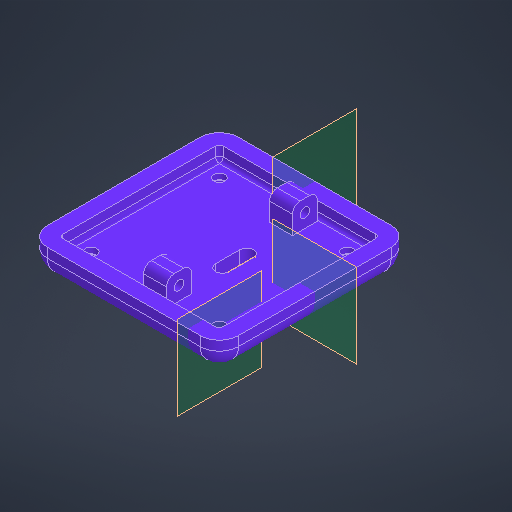
# Autodesk Inventor part: case2
Saved by Autodesk Inventor 2026.2 (Build 302298000, 298)
## iProperties
Created: 2025-11-11
Part Number: case2
Material: Generic
Document SubType Name: Modeling
Designer: micyg
Density: 1 g/cm^3
Appearance: Default
Author: micyg
Autodesk Inventor part; units mm, degrees
note: some values were not read from the file. Left out: dimensions or parameters whose unit could not be read.
ref_plane "YZ Plane" through (0, 0, 0) normal (1, 0, 0) x (0, 1, 0)
ref_plane "XZ Plane" through (0, 0, 0) normal (0, 1, 0) x (-1, 0, 0)
ref_plane "XY Plane" through (0, 0, 0) normal (0, 0, 1) x (1, 0, 0)
sketch "Sketch1" plane through (0, 0, 0) normal (0, 1, 0) x (-1, 0, 0)
  line L0 (0, 0) -> (50, 0)
  line L1 (50, 0) -> (50, -50)
  line L2 (50, -50) -> (0, -50)
  line L3 (0, -50) -> (0, 0)
  dimension "d0" = 50
  dimension "d1" = 50
  constraints: 8 end point, 2 parallel, 1 horizontal, 1 perpendicular
  measures "d0" distance of L1.end L2.end
  measures "d1" distance of L0.end L1.end
extrude "Extrusion1" add sketch "Sketch1" along normal blind 7.5
fillet "Fillet1" radius 5 4 edges at (-50, 3.75, 0) (-50, 3.75, -50) (0, 3.75, -50) (0, 3.75, 0)
ref_plane "Work Plane2" through (-25, 7.5, -50) normal (-1, 0, 0) x (0, -1, 0)
ref_plane "Work Plane1" through (0, 7.5, -25) normal (0, 0, -1) x (-1, 0, 0)
fillet "Fillet2" radius 5 8 edges at (-1.4645, 0, -48.5355) (-25, 0, -50) (-48.5355, 0, -48.5355) (-50, 0, -25) (-48.5355, 0, -1.4645) (-25, 0, 0) (-1.4645, 0, -1.4645) (0, 0, -25)
shell "Shell1" thickness 4 removed faces 1 at (-16.6667, 7.5, -18.3333)
sketch "Sketch2" plane through (0, 0, 0) normal (0, -1, 0) x (1, 0, 0)
  line L0 (-25, -60) -> (-25, 10) projected
  line L1 (10, -25) -> (-60, -25) projected
  line L2 (-8.2, -8.2) -> (-41.8, -8.2) construction
  line L3 (-41.8, -8.2) -> (-41.8, -41.8) construction
  line L4 (-41.8, -41.8) -> (-8.2, -41.8) construction
  line L5 (-8.2, -41.8) -> (-8.2, -8.2) construction
  circle A0 centre (-8.2, -8.2) radius 1.5
  point P0 (0, 0)
  point P1 (-5, -45)
  point P2 (-45, -45)
  point P3 (-25, -41.8)
  point P4 (-8.2, -25)
  point P5 (-8.2, -25)
  point P6 (-25, -41.8)
  dimension "d8" = 33.6
  dimension "d9" = 33.6
  dimension "d10" = 3
  constraints: 8 end point, 4 point on line, 2 midpoint, 2 parallel, 1 centre point, 1 coincident, 1 horizontal, 1 perpendicular
  measures "d8" distance of L4.end L2.start
  measures "d9" distance of L3.end L4.end
  measures "d10" diameter of A0
extrude "Extrusion2" cut sketch "Sketch2" against normal up to surface (4 mm away)
ref_plane "Work Plane3" through (-8.2, 0, -8.2) normal (-1, 0, 0) x (0, -1, 0)
sketch "Sketch3" plane through (-8.2, 0, -8.2) normal (-1, 0, 0) x (0, -1, 0)
  line L0 (-4, -1.5) -> (-4, 1.5) projected
  line L1 (0, 1.5) -> (0, -1.5) projected
  line L2 (0, -36.8) -> (0, 3.2) projected
  line L3 (0, 2.75) -> (-1.5, 2.75)
  line L4 (-1.5, 2.75) -> (-1.5, -2.75)
  line L5 (-1.5, -2.75) -> (0, -2.75)
  line L6 (0, -2.75) -> (0, 2.75)
  line L7 (-1.5, -2.75) -> (-2.5, -1.5)
  line L8 (0, -1.5) -> (-4, -1.5) projected
  line L9 (0, 0) -> (-4, 0)
  point P0 (0, 8.2)
  point P1 (0, -2.75)
  dimension "d13" = 5.5
  dimension "d14" = 1.5
  dimension "d15" = 1
  constraints: 12 end point, 3 midpoint, 2 parallel, 2 point on line, 1 horizontal, 1 perpendicular
  measures "d13" distance of L3.end L4.end
  measures "d14" distance of L4.end L5.end
  measures "d15" distance from line of L4 L7.end
revolve "Revolution1" cut sketch "Sketch3" angle 360 about axis through (-8.2, 0, -8.2) along (0, 1, 0) contours L8 L4 L7 | L4 L8 L2 L5
mirror "Mirror1" about plane through (0, 7.5, -25) normal (0, 0, -1) of "Extrusion2", "Revolution1"
mirror "Mirror2" about plane through (-25, 7.5, -50) normal (-1, 0, 0) of "Extrusion2", "Mirror1", "Revolution1"
sketch "Sketch4" plane through (-45, 4, -45) normal (0, 1, 0) x (1, 0, 0)
  line L0 (20, -55) -> (20, 15) construction
  line L1 (-15, -20) -> (55, -20) construction
  line L2 (24, -23.2) -> (24, -16.8) construction
  line L3 (25.8, -23.2) -> (25.8, -16.8)
  line L4 (22.2, -16.8) -> (22.2, -23.2)
  arc A0 (22.2, -23.2) -> (25.8, -23.2) centre (24, -23.2) ccw
  arc A1 (25.8, -16.8) -> (22.2, -16.8) centre (24, -16.8) ccw
  point P0 (45, -45)
  point P1 (24, -20)
  point P2 (24, -15)
  point P3 (24, -25)
  dimension "d17" = 3.6
  dimension "d38" = 6.4
  dimension "d39" = 4
  constraints: 8 end point, 6 point on circle, 4 tangent, 2 centre point, 2 parallel, 1 midpoint, 1 point on line
  measures "d17" distance between parallel lines of L3 L4
  measures "d38" distance of L2.start L2.end
  measures "d39" distance between parallel lines of L2 L0
extrude "Extrusion3" cut sketch "Sketch4" against normal up to surface (4 mm away)
ref_plane "Płaszczyzna konstrukcyjna9" through (-19.09, 4, -28.2) normal (-1, 0, 0) x (0, 0, 1)
sketch "Szkic6" plane through (-19.09, 4, -28.2) normal (-1, 0, 0) x (0, 0, 1)
  line L0 (0, 0) -> (0, 0) projected
  line L1 (0, 0) -> (6.4, 0) projected
  line L2 (6.4, 0) -> (6.4, 0) projected
  line L3 (6.4, 0) -> (0, 0) projected
  line L4 (-15.1, 0) -> (-12.1, 0) projected
  line L5 (18.5, 0) -> (21.5, 0) projected
  line L6 (-15.1, 0) -> (-12.1, 0) projected
  line L7 (18.5, 0) -> (21.5, 0) projected
  line L8 (23.2, 0) -> (-16.8, 0) projected
  line L9 (-16.8, 0) -> (23.2, 0) projected
  line L10 (6.4, -4) -> (6.4, -4) projected
  line L11 (6.4, 0) -> (6.4, -4) projected
  line L12 (6.4, 0) -> (6.4, 0) projected
  line L13 (6.4, 0) -> (6.4, -4) projected
  line L14 (0, -4) -> (0, -4) projected
  line L15 (0, 0) -> (0, -4) projected
  line L16 (0, 0) -> (0, 0) projected
  line L17 (0, 0) -> (0, -4) projected
  line L18 (-16.55, 0) -> (-10.05, 0)
  line L19 (-10.05, 0) -> (-10.05, 6.85)
  line L20 (-10.05, 6.85) -> (-16.55, 6.85)
  line L21 (-16.55, 6.85) -> (-16.55, 0)
  circle A0 centre (-13.3, 3.6) radius 1.25
  line L22 (-13.3, 0) -> (-13.3, 6.85) construction
  line L23 (3.2, -6.17) -> (3.2, 9.02) construction
  line L24 (22.95, 0) -> (16.45, 0)
  line L25 (16.45, 0) -> (16.45, 6.85)
  line L26 (16.45, 6.85) -> (22.95, 6.85)
  line L27 (22.95, 6.85) -> (22.95, 0)
  circle A1 centre (19.7, 3.6) radius 1.25
  line L28 (19.7, 0) -> (19.7, 6.85) construction
  point P0 (28.2, -4)
  point P1 (16.45, 0)
  point P2 (18.5, 0)
  point P3 (21.5, 0)
  point P4 (-16.55, 0)
  point P5 (-15.1, 0)
  point P6 (-12.1, 0)
  point P7 (-10.05, 0)
  dimension "d30" = 2
  dimension "d31" = 2
  dimension "d33" = 3.6
  dimension "d34" = 2.5
  dimension "d35" = 33
  constraints: 20 end point, 7 symmetric about line, 3 point on line, 2 centre point, 2 midpoint, 2 parallel, 1 horizontal, 1 perpendicular, 1 other
  measures "d30" distance edge to line of A0 L19
  measures "d31" distance edge to line of A0 L20
  measures "d33" distance from line of L8 A0.centre
  measures "d34" diameter of A0
  measures "d35" distance between parallel lines of L28 L22
extrude "Wyciągnięcie proste5" add sketch "Szkic6" along normal blind 6
fillet "Zaokrąglenie3" radius 2 4 edges at (-22.09, 10.85, -38.25) (-22.09, 10.85, -44.75) (-22.09, 10.85, -11.75) (-22.09, 10.85, -5.25)
equation "\"d0\" = blob_overall"
equation "\"d1\" = blob_overall"
equation "\"d4\" = corner_round"
equation "\"d5\" = corner_round"
equation "\"d6\" = shell_width"
equation "\"d31\" = d30"
equation "\"blob_overall\" = 50"
equation "\"corner_round\" = 5"
equation "\"matrix_size\" = 32"
equation "\"shell_width\" = 4"
body "Solid1"
